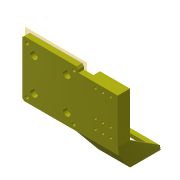
# Autodesk Inventor part: cellSTORM_v5_laserstage
Saved by Autodesk Inventor 2019 (Build 230136000, 136)
## iProperties
Created: 2020-04-25
Part Number: cellSTORM_v5_laserstage
Material: Generic
Document SubType Name: Modeling
Designer: diederichbenedict
Density: 1 g/cm^3
Appearance: Yellow
Author: diederichbenedict
Autodesk Inventor part; units mm, degrees
ref_plane "YZ Plane" through (0, 0, 0) normal (1, 0, 0) x (0, 1, 0)
ref_plane "XZ Plane" through (0, 0, 0) normal (0, 1, 0) x (-1, 0, 0)
ref_plane "XY Plane" through (0, 0, 0) normal (0, 0, 1) x (1, 0, 0)
ref_plane "Work Plane1" through (0, 0, 0) normal (0, 0, 1) x (1, 0, 0)
ref_plane "Work Plane2" through (-30, -30, 6) normal (0, 0, -1) x (0, 1, 0)
sketch "Sketch1" plane through (0, 0, 0) normal (0, 0, 1) x (1, 0, 0)
  circle A0 centre (-25, 0) radius 1.95 projected
  circle A1 centre (0, -25) radius 1.95 projected
  circle A2 centre (25, -25) radius 1.95 projected
  circle A3 centre (-25, 25) radius 1.95 projected
  circle A4 centre (25, 25) radius 1.95 projected
  circle A5 centre (-25, -25) radius 1.95 projected
  circle A6 centre (0, 25) radius 1.95 projected
  circle A7 centre (25, 0) radius 1.95 projected
  line L0 (-30, -28) -> (-28, -30) projected
  line L1 (-28, -30) -> (28, -30) projected
  line L2 (28, -30) -> (30, -28) projected
  line L3 (30, -28) -> (30, 28) projected
  line L4 (30, 28) -> (28, 30) projected
  line L5 (28, 30) -> (-28, 30) projected
  line L6 (-28, 30) -> (-30, 28) projected
  line L7 (-30, 28) -> (-30, -28) projected
  circle A8 centre (56, -8) radius 1.4 projected
  circle A9 centre (64, -8) radius 1.4 projected
  circle A10 centre (48, -8) radius 1.4 projected
  circle A11 centre (56, 20) radius 1.4 projected
  circle A12 centre (64, 20) radius 1.4 projected
  circle A13 centre (48, 20) radius 1.4 projected
  circle A14 centre (64, -18) radius 1.4 projected
  circle A15 centre (56, -18) radius 1.4 projected
  circle A16 centre (48, -18) radius 1.4 projected
  line L8 (40, 25) -> (72, 25) projected
  line L9 (40, 25) -> (40, -23) projected
  line L10 (72, -23) -> (40, -23) projected
  line L11 (72, 25) -> (72, -23) projected
  line L12 (40, 25) -> (30, 25)
  line L13 (66.4723, -44) -> (76, -44) projected
  line L14 (72, -23) -> (76, -44)
  line L15 (76, -44) -> (42, -44)
  line L16 (42, -44) -> (28, -30)
  line L17 (43, -44) -> (44, -44) projected
  point P0 (0, 0)
  constraints: 8 end point, 1 horizontal, 1 perpendicular, 1 point on line
extrude "Extrusion1" add sketch "Sketch1" along normal up to surface (6 mm away) contours A0 | A1 | A2 | A3 | A4 | A5 | A6 | A7 | L7 L6 L5 L4 L3 L2 L1 L0 | L2 L3 L12 L9 L10 L14 L13 L15 L16 | L8 L11 L10 L9
sketch "Sketch2" plane through (-28, 30, 6) normal (0, 0, 1) x (1, 0, 0)
  circle A0 centre (10.5, -12.5) radius 1.95 projected
  circle A1 centre (10.5, -47.5) radius 1.95 projected
  circle A2 centre (45.5, -47.5) radius 1.95 projected
  circle A3 centre (45.5, -12.5) radius 1.95 projected
  point P0 (28, -30)
hole "Hole1" at (-17.5, -17.5, 6) at (17.5, -17.5, 6) at (17.5, 17.5, 6) at (-17.5, 17.5, 6) direction (0, 0, -1) diameter 4 end through all counterbore diameter 8 counterbore depth 4.5
sketch "Sketch4" plane through (0, 0, 0) normal (0, 0, -1) x (-1, 0, 0)
  line L0 (-28, -30) -> (-42, -44) projected
  line L1 (-42, -44) -> (-76, -44) projected
  line L2 (-76, -44) -> (-72, -23) projected
  line L3 (-75.2381, -40) -> (-38, -40)
  line L4 (-72, -40) -> (-71.746, -39.8945)
  point P0 (0, 0)
  dimension "d16" = 4
  constraints: 4 end point, 3 point on line, 1 horizontal, 1 parallel
  measures "d16" distance between parallel lines of L1 L3
extrude "Extrusion2" add sketch "Sketch4" along normal up to surface (35.7 mm away)
sketch "Sketch5" plane through (72, -23, 6) normal (0.9823386, 0.1871121, 0) x (0, 0, -1)
  line L0 (0, -21.3776) -> (0, 0) projected
  line L1 (41.7, -21.3776) -> (0, -21.3776) projected
  line L2 (41.7, -21.3776) -> (41.7, -17.3056) projected
  line L3 (6, -17.3056) -> (41.7, -17.3056) projected
  line L4 (6, -17.3056) -> (6, 0) projected
  line L5 (6, 0) -> (0, 0) projected
  line L6 (13, 47.1523) -> (13, 0) projected
  line L7 (6, 0) -> (13, 0)
  line L8 (13, 0) -> (41.7, -17.3056)
  point P0 (6, 36.0659)
  point P1 (41.3101, -17.3056)
  constraints: 4 end point, 1 perpendicular, 1 point on line
extrude "Extrusion3" add sketch "Sketch5" against normal blind 4
sketch "Sketch6" plane through (42, -44, 6) normal (0, -1, 0) x (1, 0, 0)
  arc A0 (29.8555, -40.7) -> (30.8555, -41.7) centre (30.8555, -40.7) ccw construction
  line L0 (30.8555, -41.7) -> (34, -41.7) construction
  line L1 (34, -41.7) -> (34, -16) construction
  line L2 (34, -16) -> (24.4723, -16) construction
  arc A1 (24.4723, -16) -> (23.4723, -17) centre (24.4723, -17) ccw construction
  line L3 (23.4723, -17) -> (23.4723, -18.8624) construction
  arc A2 (22.4723, -19.8624) -> (23.4723, -18.8624) centre (22.4723, -18.8624) ccw construction
  line L4 (22.4723, -19.8624) -> (4, -19.8624) construction
  line L5 (4, -19.8624) -> (4, -31.397) construction
  arc A3 (3, -32.397) -> (4, -31.397) centre (3, -31.397) ccw construction
  line L6 (3, -32.397) -> (2, -32.397) construction
  arc A4 (2, -32.397) -> (1, -33.397) centre (2, -33.397) ccw construction
  line L7 (1, -33.397) -> (1, -35.9624) construction
  arc A5 (1, -35.9624) -> (2, -36.9624) centre (2, -35.9624) ccw construction
  line L8 (2, -36.9624) -> (28.8555, -36.9624) construction
  arc A6 (29.8555, -37.9624) -> (28.8555, -36.9624) centre (28.8555, -37.9624) ccw construction
  line L9 (29.8555, -37.9624) -> (29.8555, -40.7) construction
  line L10 (21.5, -35) -> (6, -35) construction
  line L11 (6, -35) -> (6, -21.5) construction
  line L12 (6, -21.5) -> (21.5, -21.5) construction
  line L13 (21.5, -21.5) -> (21.5, -35) construction
  circle A7 centre (31.5, -39) radius 1 construction
  circle A8 centre (25, -18.5) radius 1 construction
  circle A9 centre (3.5, -34) radius 1 construction
  line L14 (6, -21.5) -> (21.5, -21.5) construction
  line L15 (21.5, -21.5) -> (21.5, -35) construction
  line L16 (21.5, -35) -> (6, -35) construction
  line L17 (6, -35) -> (6, -21.5) construction
  line L18 (6, -21.5) -> (21.5, -21.5)
  line L19 (21.5, -21.5) -> (21.5, -35)
  line L20 (21.5, -35) -> (6, -35)
  line L21 (6, -35) -> (6, -21.5)
  circle A10 centre (25, -18.5) radius 1
  circle A11 centre (31.5, -39) radius 1
  circle A12 centre (3.5, -34) radius 1
  line L22 (5.1585, -23.6778) -> (27.4978, -23.6778)
  line L23 (27.4978, -23.6778) -> (27.4978, -36.9624)
  line L24 (27.4978, -36.9624) -> (5.1585, -36.9624)
  line L25 (5.1585, -36.9624) -> (5.1585, -23.6778)
  point P0 (-42, -6)
  constraints: 24 end point, 6 parallel, 3 centre point, 3 coincident, 3 concentric, 3 horizontal, 3 perpendicular, 1 point on line
extrude "Extrusion4" cut sketch "Sketch6" against normal through all
sketch "Sketch7" plane through (0, 0, 0) normal (0, 0, -1) x (-1, 0, 0)
  circle A0 centre (-56, -8) radius 1.4 projected
  circle A1 centre (-64, -8) radius 1.4 projected
  circle A2 centre (-48, -8) radius 1.4 projected
  circle A3 centre (-56, 20) radius 1.4 projected
  circle A4 centre (-64, 20) radius 1.4 projected
  circle A5 centre (-48, 20) radius 1.4 projected
  circle A6 centre (-64, -18) radius 1.4 projected
  circle A7 centre (-56, -18) radius 1.4 projected
  circle A8 centre (-48, -18) radius 1.4 projected
  line L0 (-40, 25) -> (-72, 25) projected
  line L1 (-40, 25) -> (-40, -23) projected
  line L2 (-72, -23) -> (-40, -23) projected
  line L3 (-72, 25) -> (-72, -23) projected
  arc A9 (-49, 2.2984) -> (-49, 0.7016) centre (-47.85, 1.5) ccw
  arc A10 (-63, 2.2984) -> (-63, 0.7016) centre (-64.15, 1.5) ccw
  arc A11 (-49, 0.7016) -> (-49, 2.2984) centre (-47.85, 1.5) ccw
  circle A12 centre (-47.85, 1.5) radius 1.4
  circle A13 centre (-64.15, 1.5) radius 1.4
  point P0 (0, 0)
  constraints: 6 point on circle, 5 centre point, 2 coincident, 2 concentric, 10 other
ref_plane "Work Plane3" through (40, -23, -7) normal (0, 0, 1) x (1, 0, 0)
extrude "Extrusion5" add sketch "Sketch7" along normal up to surface (7 mm away) contours L1 L2 L3 L0 | A11 A9 | A13 A10
sketch "Sketch8" plane through (72, -23, 6) normal (1, 0, 0) x (0, 0, -1)
  line L0 (0, -21) -> (0, 0) projected
  line L1 (41.7, -21) -> (0, -21) projected
  line L2 (41.7, -21) -> (41.7, -17) projected
  line L3 (41.7, -17) -> (13, 0) projected
  line L4 (13, 0) -> (6, 0) projected
  line L5 (6, 0) -> (0, 0) projected
  line L6 (-8, -7) -> (0, -7) projected
  line L7 (0, -7) -> (9.1538, -21)
  line L8 (41.7, -21) -> (0, -21) projected
  line L9 (0, -21) -> (9.1538, -21)
  line L10 (0, -21) -> (0, -7)
  line L11 (0, -7) -> (0, -21) projected
  line L12 (0, -21) -> (41.7, -21)
  line L13 (41.7, -21) -> (41.7, -23.7437)
  line L14 (41.7, -23.7437) -> (0, -23.7437)
  line L15 (0, -23.7437) -> (0, -21)
  point P0 (6, 23)
  constraints: 14 end point, 2 horizontal, 2 parallel, 2 perpendicular, 1 point on line
extrude "Extrusion6" cut sketch "Sketch8" along normal through all both and the other way through all contours L0 L7 L1 | L1 L13 L14 L15
sketch "Sketch9" plane through (40, -23, 0) normal (-1, 0, 0) x (0, 0, 1)
  line L0 (-0.5384, -17) -> (0, -16.1766) projected
  line L1 (0, -0.7484) -> (0, -16.1766) projected
  line L2 (0, -0.7484) -> (-7, -0.7484) projected
  line L3 (-7, -0.7484) -> (-17.6778, -7.0733) projected
  line L4 (-17.6778, -7.0733) -> (-17.6778, -8.2408) projected
  line L5 (-17.6778, -8.2408) -> (-19.6488, -8.2408) projected
  line L6 (-19.6488, -8.2408) -> (-34.4364, -17) projected
  line L7 (-0.5384, -17) -> (-34.4364, -17) projected
  line L8 (-0.5384, -17) -> (-34.4364, -17) projected
  line L9 (-4.1227, -17) -> (0, -10.6946)
  line L10 (0, -0.7484) -> (0, -16.1766) projected
  point P0 (0, 23)
  dimension "d29" = 3
  constraints: 2 end point, 2 point on line, 1 parallel
  measures "d29" distance between parallel lines of L9 L0
extrude "Extrusion7" add sketch "Sketch9" along normal up to surface contours L7 L9 L1 L0 starts on plane at (70.987, -39.0592, -9.9528) facing (-0.9823386, -0.1871121, 0) surface through (28, -30, 0) normal (-0.7071068, -0.7071068, 0)
sketch "Sketch10" plane through (0, 0, 0) normal (0, 0, -1) x (-1, 0, 0)
  circle A0 centre (-25, 25) radius 2.325 projected
  circle A1 centre (-25, -25) radius 2.325 projected
  circle A2 centre (25, 25) radius 2.325 projected
  circle A3 centre (25, -25) radius 2.325 projected
  circle A4 centre (25, -25) radius 2.325 projected
  point P0 (0, 0)
hole "Hole3" at (-25, 25, 0) at (25, 25, 0) at (-25, -25, 0) at (25, -25, 0) direction (0, 0, 1) diameter 3.8 depth 20 tip angle 118
body "Solid1"
